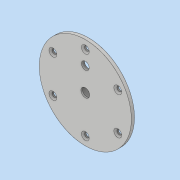
# Autodesk Inventor part: SpoolEndFrontSide
Saved by Autodesk Inventor 2017 (Build 210142000, 142)
## iProperties
Created: 2016-11-06
Part Number: SpoolEndFrontSide
Material: Generic
Document SubType Name: Modeling
Designer: techn
Density: 1 g/cm^3
Appearance: Default
Author: techn
Autodesk Inventor part; units mm, degrees
ref_plane "YZ Plane" through (0, 0, 0) normal (1, 0, 0) x (0, 1, 0)
ref_plane "XZ Plane" through (0, 0, 0) normal (0, 1, 0) x (-1, 0, 0)
ref_plane "XY Plane" through (0, 0, 0) normal (0, 0, 1) x (1, 0, 0)
sketch "Sketch1" plane through (0, 0, 0) normal (0, 0, 1) x (1, 0, 0)
  circle A0 centre (0, 0) radius 37.465
  dimension "d0" = 74.93
  constraints: 1 centre point, 1 coincident
  measures "d0" diameter of A0
extrude "Extrusion1" add sketch "Sketch1" along normal blind 2.54
sketch "Sketch3" plane through (0, 0, 0) normal (0, 0, -1) x (-1, 0, 0)
  circle A0 centre (0, 0) radius 4.191
  circle A1 centre (0, 0) radius 7.9375
  circle A2 centre (0, 0) radius 2.3813
  dimension "d4" = 8.382
  dimension "d5" = 15.875
  dimension "d6" = 4.7625
  constraints: 3 centre point, 3 coincident
  measures "d4" diameter of A0
  measures "d5" diameter of A1
  measures "d6" diameter of A2
extrude "Extrusion3" cut sketch "Sketch3" against normal through all contours A0 | A2
extrude "Extrusion4" add sketch "Sketch3" along normal blind 5.08 contours A1
sketch "Sketch4" plane through (0, 0, 2.54) normal (0, 0, 1) x (1, 0, 0)
  line L0 (0, 0) -> (0, 30.48)
  circle A0 centre (0, 30.48) radius 1.905
  circle A1 centre (-26.3965, 15.24) radius 1.905
  circle A2 centre (-26.3965, -15.24) radius 1.905
  circle A3 centre (0, -30.48) radius 1.905
  circle A4 centre (26.3965, -15.24) radius 1.905
  circle A5 centre (26.3965, 15.24) radius 1.905
  dimension "d13" = 30.48
  dimension "d14" = 3.81
  dimension "d17" = 360
  constraints: 6 centre point, 2 end point, 1 coincident, 1 vertical, 13 other
  measures "d13" distance of L0.start L0.end
  measures "d14" diameter of A0
extrude "Extrusion5" cut sketch "Sketch4" against normal blind 25.4
sketch "Sketch6" plane through (0, 0, 2.54) normal (0, 0, 1) x (1, 0, 0)
  circle A0 centre (0, 0) radius 3.556
  circle A1 centre (0, 0) radius 4.191 projected
  dimension "d21" = 7.112
  constraints: 1 centre point, 1 coincident
  measures "d21" diameter of A0
extrude "Extrusion6" add sketch "Sketch6" against normal blind 1.27
chamfer "Chamfer1" distance 1.27 angle 45 6 edges at (-28.3015, -15.24, 2.54) (-28.3015, 15.24, 2.54) (-1.905, 30.48, 2.54) (-1.905, -30.48, 2.54) (24.4915, -15.24, 2.54) (24.4915, 15.24, 2.54)
sketch "Sketch7" plane through (0, 0, 2.54) normal (0, 0, 1) x (1, 0, 0)
  circle A0 centre (0, 19.05) radius 3.175
  point P0 (0, 0)
  dimension "d27" = 6.35
  dimension "d28" = 19.05
  constraints: 1 centre point
  measures "d27" diameter of A0
  measures "d28" distance of point (0, 0) A0.centre
extrude "Extrusion7" cut sketch "Sketch7" against normal through all
body "Solid1"
